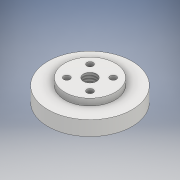
# Autodesk Inventor part: Ground_Tracker_TripodMount
Saved by Autodesk Inventor 2018 (Build 220112000, 112)
## iProperties
Created: 2018-09-27
Part Number: Ground_Tracker_TripodMount
Material: UHMW, White
Document SubType Name: Modeling
Designer: Bradley
Density: 0.94 g/cm^3
Appearance: Smooth - White
Author: Bradley
Autodesk Inventor part; units mm, degrees
ref_plane "YZ Plane" through (0, 0, 0) normal (1, 0, 0) x (0, 1, 0)
ref_plane "XZ Plane" through (0, 0, 0) normal (0, 1, 0) x (-1, 0, 0)
ref_plane "XY Plane" through (0, 0, 0) normal (0, 0, 1) x (1, 0, 0)
sketch "Sketch1" plane through (0, 0, 0) normal (0, 1, 0) x (-1, 0, 0)
  line L0 (0, 6.35) -> (-15, 6.35)
  line L1 (-15, 6.35) -> (-15, 2.35)
  line L2 (-15, 2.35) -> (-25, 2.35)
  line L3 (-25, 2.35) -> (-25, -6.35)
  line L4 (-25, -6.35) -> (0, -6.35)
  line L5 (0, -6.35) -> (0, 6.35)
  point P0 (0, 0)
  point P1 (0, 0)
  dimension "d0" = 30
  dimension "d1" = 10
  dimension "d2" = 12.7
  dimension "d3" = 4
  constraints: 12 end point, 5 perpendicular, 1 coincident, 1 horizontal, 1 midpoint
  measures "d0" diameter of L1 L5
  measures "d1" distance of L1.end L2.end
  measures "d2" distance of L4.end L0.start
  measures "d3" distance of L0.end L1.end
revolve "Revolution1" add sketch "Sketch1" angle 360 about axis through (0, 0, -6.35) along (0, 0, 1)
hole "Hole1" at (0, 0, 6.35) direction (0, 0, -1) diameter 7.798 end through all thread size "3/8-16 UNC" class "2B" standard "ANSI Unified Screw Threads"
sketch "Sketch3" plane through (0, 0, -6.35) normal (0, 0, -1) x (-1, 0, 0)
  line L0 (-6.9148, 6.9148) -> (6.9148, 6.9148)
  line L1 (6.9148, 6.9148) -> (6.9148, -6.9148)
  line L2 (6.9148, -6.9148) -> (-6.9148, -6.9148)
  line L3 (-6.9148, -6.9148) -> (-6.9148, 6.9148)
  line L4 (-6.9148, 6.9148) -> (6.9148, -6.9148) construction
  line L5 (6.9148, 6.9148) -> (-6.9148, -6.9148) construction
  point P0 (0, 0)
  dimension "d14" = 19.558
  constraints: 12 end point, 4 coincident, 2 midpoint, 2 parallel, 2 perpendicular, 1 horizontal
  measures "d14" distance of L0.end L2.end
hole "Hole2" at (-6.9148, 6.9148, -6.35) at (-6.9148, -6.9148, -6.35) at (6.9148, -6.9148, -6.35) at (6.9148, 6.9148, -6.35) direction (0, 0, 1) diameter 3.797 end through all counterbore diameter 7.145 counterbore depth 3.505 clearance for "Socket Head Cap Screw" size "#6" standard "Ansi Unified Screw Threads"
body "Solid1"
